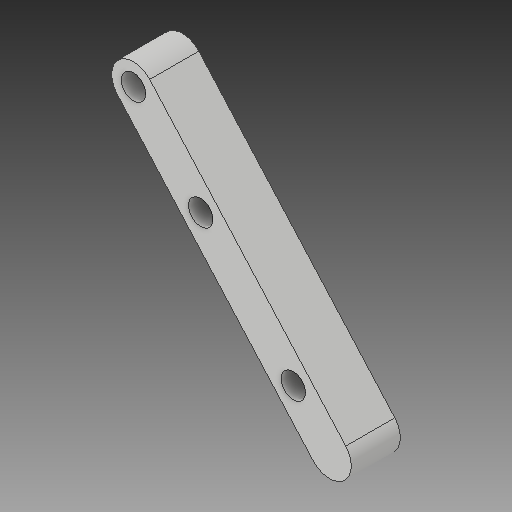
# Autodesk Inventor part: MassiveBone3
Saved by Autodesk Inventor 2017 (Build 210142000, 142)
## iProperties
Created: 2020-09-06
Part Number: MassiveBone3
Material: Generic
Document SubType Name: Modeling
Designer: agustin
Density: 1 g/cm^3
Appearance: Default
Author: agustin
Autodesk Inventor part; units mm, degrees
ref_plane "YZ Plane" through (0, 0, 0) normal (1, 0, 0) x (0, 1, 0)
ref_plane "XZ Plane" through (0, 0, 0) normal (0, 1, 0) x (-1, 0, 0)
ref_plane "XY Plane" through (0, 0, 0) normal (0, 0, 1) x (1, 0, 0)
sketch "Sketch1" plane through (0, 0, 0) normal (0, 0, 1) x (1, 0, 0)
  circle A0 centre (20.6614, -0.7818) radius 2.25 projected
  circle A1 centre (3.6717, 18.234) radius 2.25 projected
  circle A2 centre (-8.6609, 32.0238) radius 2.25 projected
  arc A3 (24.8863, -10.4155) -> (29.7342, -6.0856) centre (27.3102, -8.2505) ccw projected
  line L0 (27.3102, -8.2505) -> (-8.6609, 32.0238) construction
  line L1 (30.2936, -5.586) -> (-5.6776, 34.6883)
  line L2 (-11.6442, 29.3592) -> (24.3269, -10.9151)
  arc A4 (24.3269, -10.9151) -> (30.2936, -5.586) centre (27.3102, -8.2505) ccw
  arc A5 (-5.6776, 34.6883) -> (-11.6442, 29.3592) centre (-8.6609, 32.0238) ccw
  point P0 (0, 0)
  point P1 (9.3247, 11.8866)
  dimension "d0" = 8
  constraints: 8 end point, 4 point on circle, 4 tangent, 2 centre point, 1 midpoint, 1 parallel
  measures "d0" diameter of A5
extrude "Extrusion1" add sketch "Sketch1" along normal blind 9
scale "Scale1" factors (0.5, 0.5, 0.5) then translate (3.1707, 4.611, 2.25) bodies 1
body "Solid1"
